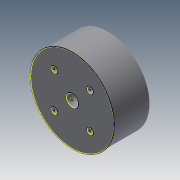
# Autodesk Inventor part: drivepulleyMiddle
Saved by Autodesk Inventor 2015 (Build 190159000, 159)
## iProperties
Created: 2014-09-01
Part Number: drivepulleyMiddle
Material: Generic
Document SubType Name: Modeling
Designer: shohei
Density: 1 g/cm^3
Appearance: Default
Author: shohei
Autodesk Inventor part; units mm, degrees
ref_plane "YZ Plane" through (0, 0, 0) normal (1, 0, 0) x (0, 1, 0)
ref_plane "XZ Plane" through (0, 0, 0) normal (0, 1, 0) x (-1, 0, 0)
ref_plane "XY Plane" through (0, 0, 0) normal (0, 0, 1) x (1, 0, 0)
sketch "Block1" plane through (0, 0, 0) normal (0, 0, 1) x (1, 0, 0)
  circle A0 centre (0, 0) radius 50.22
  circle A1 centre (-30, -32.5) radius 2.72
  circle A2 centre (30, -32.5) radius 2.72
  circle A3 centre (0, 0) radius 5.22
  circle A4 centre (-30, 32.5) radius 2.72
  circle A5 centre (30, 32.5) radius 2.72
sketch "Block2" plane through (0, 0, 0) normal (0, 0, 1) x (1, 0, 0)
  circle A0 centre (0, 0) radius 35.22
  circle A1 centre (0, 0) radius 5.22
  circle A2 centre (20, 20) radius 2.72
  circle A3 centre (-20, 20) radius 2.72
  circle A4 centre (-20, -20) radius 2.72
  circle A5 centre (20, -20) radius 2.72
  point P0 (0, 0)
sketch "Block3" plane through (0, 0, 0) normal (0, 0, 1) x (1, 0, 0)
  circle A0 centre (0, 0) radius 35.22
  circle A1 centre (-15, 17.5) radius 2.72
  circle A2 centre (0, 0) radius 5.22
  circle A3 centre (-15, -17.5) radius 2.72
  circle A4 centre (15, 17.5) radius 2.72
  circle A5 centre (15, -17.5) radius 2.72
sketch "Block4" plane through (0, 0, 0) normal (0, 0, 1) x (1, 0, 0)
  circle A0 centre (0, 0) radius 35.22
  circle A1 centre (-15, 15) radius 2.72
  circle A2 centre (-15, -15) radius 2.72
  circle A3 centre (0, 0) radius 5.22
  circle A4 centre (15, 15) radius 2.72
  circle A5 centre (15, -15) radius 2.72
sketch "Sketch1" plane through (0, 0, 0) normal (0, 1, 0) x (-1, 0, 0)
  circle A0 centre (0, 0) radius 35
  line L0 (49, 0) -> (-49, 0) projected
  line L1 (0, -49) -> (0, 49) projected
  circle A1 centre (-15, -15) radius 2.5
  circle A2 centre (15, -15) radius 2.5
  circle A3 centre (-15, 15) radius 2.5
  circle A4 centre (15, 15) radius 2.5
  circle A5 centre (0, 0) radius 5
  dimension "d0" = 70
  dimension "d29" = 5
  dimension "d30" = 15
  dimension "d31" = 15
  dimension "d34" = 10
  constraints: 6 centre point, 3 symmetric about line, 1 coincident, 3 other
  measures "d0" diameter of A0
  measures "d29" diameter of A1
  measures "d30" distance from line of L1 A1.centre
  measures "d31" distance from line of L0 A1.centre
  measures "d34" diameter of A5
extrude "Extrusion5" add sketch "Sketch1" along normal blind 30 contours L0 A5 L1 A0 | A0 L1 A5 L0 | L1 A5 L0 A0 | A0 L0 A5 L1
sketch "Sketch9" plane through (0, 0, 0) normal (0, -1, 0) x (1, 0, 0)
  circle A0 centre (0, 0) radius 5 projected
  circle A1 centre (-15, 15) radius 2.5 projected
  circle A2 centre (15, 15) radius 2.5 projected
  circle A3 centre (-15, -15) radius 2.5 projected
  circle A4 centre (15, -15) radius 2.5 projected
  circle A5 centre (0, 0) radius 35 projected
  constraints: 6 other
sketch "DXF" plane through (0, 0, 0) normal (0, 1, 0) x (-1, 0, 0)
  point P0 (0, 0)
body "Solid5"
